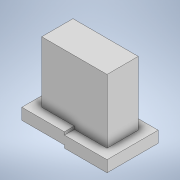
# Autodesk Inventor part: Black_Keyboard_Button_Prong
Saved by Autodesk Inventor 2021 (Build 250183000, 183)
## iProperties
Created: 2020-06-05
Part Number: Black_Keyboard_Button_Prong
Material: Generic
Document SubType Name: Modeling
Designer: ameli
Density: 1 g/cm^3
Appearance: Default
Author: ameli
Autodesk Inventor part; units mm, degrees
ref_plane "YZ Plane" through (0, 0, 0) normal (1, 0, 0) x (0, 1, 0)
ref_plane "XZ Plane" through (0, 0, 0) normal (0, 1, 0) x (-1, 0, 0)
ref_plane "XY Plane" through (0, 0, 0) normal (0, 0, 1) x (1, 0, 0)
sketch "Sketch1" plane through (0, 0, 0) normal (0, 1, 0) x (-1, 0, 0)
  line L0 (0, 0) -> (5.75, 0)
  line L1 (5.75, 0) -> (5.75, 5.5)
  line L2 (5.75, 5.5) -> (0, 5.5)
  line L3 (0, 5.5) -> (0, 0)
  point P0 (0, 0)
  dimension "d0" = 5.75
  dimension "d1" = 5.5
  dimension "d2" = 0
  dimension "d3" = 0
  constraints: 8 end point, 2 parallel, 1 horizontal, 1 perpendicular
  measures "d0" distance of L0.start L0.end
  measures "d1" distance of L0.end L1.end
  measures "d2" distance of point (0, 0) L0.start
  measures "d3" distance from line of point (0, 0) L3
extrude "Extrusion1" add sketch "Sketch1" along normal blind 10.75
sketch "Sketch2" plane through (0, 0, 5.5) normal (1, 0, 0) x (0, 0, -1)
  line L0 (5.5, 10.75) -> (0, 10.75) projected
  line L1 (0, 10.75) -> (5.5, 10.75)
  line L2 (5.5, 10.75) -> (5.5, -0.5)
  line L3 (5.5, -0.5) -> (0, -0.5)
  line L4 (0, -0.5) -> (0, 10.75)
  point P0 (5.5, 0)
  dimension "d6" = 11.25
  dimension "d7" = 5.5
  constraints: 8 end point, 2 parallel, 1 horizontal, 1 perpendicular
  measures "d6" distance of L1.end L2.end
  measures "d7" distance between parallel lines of L4 L2
extrude "Extrusion2" add sketch "Sketch2" along normal blind 5.75
sketch "Sketch3" plane through (0, -0.5, 0) normal (0, -1, 0) x (1, 0, 0)
  line L0 (0, -1.75) -> (7.5, -1.75)
  line L1 (7.5, -1.75) -> (7.5, 7.25)
  line L2 (7.5, 7.25) -> (0, 7.25)
  line L3 (0, 7.25) -> (0, -1.75)
  line L4 (0, 5.5) -> (0, 0) projected
  line L5 (0, 5.5) -> (5.75, 5.5) projected
  dimension "d10" = 9
  dimension "d11" = 7.5
  dimension "d12" = 0
  dimension "d13" = 1.75
  constraints: 8 end point, 2 parallel, 1 horizontal, 1 perpendicular
  measures "d10" distance of L0.end L1.end
  measures "d11" distance of L1.end L2.end
  measures "d12" distance between parallel lines of L4 L3
  measures "d13" distance between parallel lines of L5 L2
extrude "Extrusion3" add sketch "Sketch3" along normal blind 2
sketch "Sketch4" plane through (0, 0, 0) normal (0, -1, 0) x (1, 0, 0)
  line L0 (-7.5, 7.25) -> (0, 7.25)
  line L1 (0, 7.25) -> (0, -1.75)
  line L2 (0, -1.75) -> (-7.5, -1.75)
  line L3 (-7.5, -1.75) -> (-7.5, 7.25)
  line L4 (0, 5.5) -> (0, 0) projected
  line L5 (0, 0) -> (-5.75, 0) projected
  dimension "d16" = 9
  dimension "d17" = 7.5
  dimension "d18" = 0
  dimension "d19" = 1.75
  constraints: 8 end point, 2 parallel, 1 horizontal, 1 perpendicular
  measures "d16" distance of L2.end L0.start
  measures "d17" distance of L0.start L0.end
  measures "d18" distance between parallel lines of L4 L1
  measures "d19" distance between parallel lines of L5 L2
extrude "Extrusion4" add sketch "Sketch4" along normal blind 2
body "Solid1"
